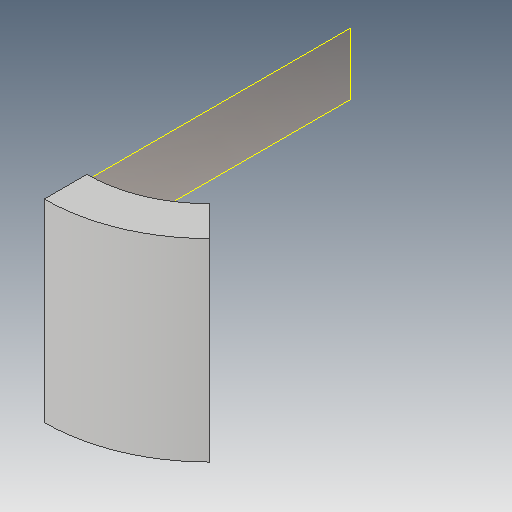
# Autodesk Inventor part: 30_CUBE_openVCM_housing_v0
Saved by Autodesk Inventor 2019 (Build 230136000, 136)
## iProperties
Created: 2020-01-31
Part Number: 30_CUBE_openVCM_housing_v0
Material: Generic
Document SubType Name: Modeling
Designer: diederichbenedict
Density: 1 g/cm^3
Appearance: Default
Author: diederichbenedict
Autodesk Inventor part; units mm, degrees
ref_plane "YZ Plane" through (0, 0, 0) normal (1, 0, 0) x (0, 1, 0)
ref_plane "XZ Plane" through (0, 0, 0) normal (0, 1, 0) x (-1, 0, 0)
ref_plane "XY Plane" through (0, 0, 0) normal (0, 0, 1) x (1, 0, 0)
ref_plane "Work Plane1" through (-78.4021, 45.2937, 54.7847) normal (1, 0, 0) x (0, -1, 0)
sketch "Sketch1" plane through (-78.4021, 45.2937, 54.7847) normal (1, 0, 0) x (0, -1, 0)
  line L0 (-10.7249, -24.5087) -> (-6.2749, -24.5087) construction
  line L1 (-10.7249, 24.5087) -> (-10.7249, -24.5087) construction
  line L2 (-6.2749, -24.5087) -> (-6.2749, 24.5087) construction
  line L3 (0, 30) -> (0, -30) construction
  line L4 (10, -30) -> (10, 30) construction
  line L5 (10, -30) -> (0, -30) construction
  line L6 (18.7251, 24.5087) -> (18.7251, -24.5087) construction
  line L7 (23.1751, -24.5087) -> (23.1751, 24.5087) construction
  line L8 (23.1751, -24.5087) -> (18.7251, -24.5087) construction
  line L9 (-57.6887, 0) -> (62.4574, 0) construction
  line L10 (-11.2249, 24.5087) -> (-11.2249, -25.0087) construction
  line L11 (-11.2249, -25.0087) -> (-5.7749, -25.0087) construction
  line L12 (-5.7749, -25.0087) -> (-5.7749, 24.5087) construction
  line L13 (-0.5, 30) -> (-0.5, -30.5) construction
  line L14 (-0.5, -30.5) -> (10.5, -30.5) construction
  line L15 (10.5, -30.5) -> (10.5, 30) construction
  line L16 (18.2251, 24.5087) -> (18.2251, -25.0087) construction
  line L17 (18.2251, -25.0087) -> (23.6751, -25.0087) construction
  line L18 (23.6751, -25.0087) -> (23.6751, 24.5087) construction
  line L19 (-11.2249, -23.3773) -> (-12.2249, -23.3773)
  line L20 (-12.2249, -23.3773) -> (-12.2249, -31.5213)
  line L21 (23.6751, -23.3773) -> (24.6751, -23.3773)
  line L22 (24.6751, -23.3773) -> (24.6751, -31.5213)
  line L23 (24.6751, -31.5213) -> (-12.2249, -31.5213)
  line L24 (23.6751, -23.3773) -> (23.6751, -25.0087)
  line L25 (23.6751, -25.0087) -> (18.2251, -25.0087)
  line L26 (18.2251, -25.0087) -> (18.2251, -23.3773)
  line L27 (18.2251, -23.3773) -> (10.5, -28.7955)
  line L28 (10.5, -28.7955) -> (10.5, -30.5)
  line L29 (10.5, -30.5) -> (-0.5, -30.5)
  line L30 (-5.7749, -23.3773) -> (-5.7749, -25.0087)
  line L31 (-5.7749, -25.0087) -> (-11.2249, -25.0087)
  line L32 (-11.2249, -23.3773) -> (-11.2249, -25.0087)
  line L33 (-0.5, -30.5) -> (-0.5, -28.7955)
  line L34 (-0.5, -28.7955) -> (-5.7749, -23.3773)
  point P0 (45.2937, 54.7847)
  dimension "d0" = 0.5
  dimension "d1" = 0.5
  dimension "d2" = 0.5
  dimension "d3" = 1
  dimension "d4" = 1
  constraints: 58 end point, 7 point on line, 6 perpendicular, 5 horizontal, 3 collinear, 1 vertical, 10 other
  measures "d0" distance between parallel lines of L1 L10
  measures "d1" distance between parallel lines of L5 L14
  measures "d2" distance between parallel lines of L6 L16
  measures "d3" distance of L19.start L19.end
  measures "d4" distance of L21.start L21.end
revolve "Revolution1" add sketch "Sketch1" angle 45 about axis through (-78.4021, 102.9823, 54.7847) along (0, 1, 0)
body "Solid1"
